lamp2 (Autodesk Fusion 360 design; units mm, degrees)
Autodesk Fusion 360 part; units mm, degrees
note: some values were not read from the file. Set by a fixed rule: which sketch regions a step uses.
sketch "Sketch1" plane through (0, 0, 0) normal (0, 0, 1) x (1, 0, 0)
  circle A0 centre (0, 0) radius 26
  circle A1 centre (0, 0) radius 16.5
  dimension "d1" = 52
  dimension "d2" = 33
  constraint coincident A0.centre A1.centre
  measures "d1" diameter of A0
  measures "d2" diameter of A1
extrude "Extrude1" add sketch "Sketch1" along normal blind 10 makes body 1
sketch "Sketch2" plane through (0, 0, 0) normal (0, 0, -1) x (1, 0, 0)
  circle A0 centre (0, 0) radius 16.5
  circle A1 centre (0, 0) radius 26
  circle A2 centre (0, 0) radius 20.5
  circle A3 centre (0, 0) radius 26
  dimension "d5" = 41
  constraint coincident A0.centre A1.centre
  constraint concentric A2 A3
  measures "d5" diameter of A2
extrude "Extrude2" add sketch "Sketch2" along normal blind 20 contours A1 A3 bodies 1
sketch "Sketch3" plane through (0, 0, -20) normal (0, 0, -1) x (1, 0, 0)
  circle A0 centre (0, 0) radius 20.5
  circle A1 centre (0, 0) radius 26
  circle A2 centre (0, 0) radius 26
  circle A3 centre (0, 0) radius 22
  dimension "d8" = 44
  constraint coincident A0.centre A1.centre
  constraint concentric A2 A3
  measures "d8" diameter of A3
extrude "Extrude3" add sketch "Sketch3" along normal blind 60 contours A1 A2 bodies 1
sketch "Sketch4" plane through (0, 0, 0) normal (0, 1, 0) x (1, 0, 0)
  circle A0 centre (0, 76) radius 4
  line L0 (0, 87) -> (0, 61.5698)
  line L1 (-16, 80) -> (14, 80)
  line L2 (-4, 76) -> (4, 76)
  line L3 (4, 76) -> (4, 83.4251)
  line L4 (4, 83.4251) -> (-4, 83.4251)
  line L5 (-4, 83.4251) -> (-4, 76)
  point P0 (0, 80)
  dimension "d11" = 8
  dimension "d12" = 8
  constraint vertical L0
  constraint horizontal L1
  constraint tangent A0 L1
  constraint coincident A0.centre L0
  constraint coincident L1 P0
  constraint coincident L0 P0
  constraint horizontal L2
  constraint vertical L3
  constraint horizontal L4
  constraint vertical L5
  constraint coincident A0.centre L2
  constraint coincident A0 L2.start
  measures "d11" diameter of A0
  measures "d12" distance of L2.start L2.end
extrude "Extrude4" cut sketch "Sketch4" along normal blind 70 bodies 1
sketch "Sketch5" plane through (0, 0, -80) normal (0, 0, -1) x (1, 0, 0)
  line L0 (-4, -25.6905) -> (-4, -21.6333)
  arc A0 (4, -21.6333) -> (-4, -21.6333) centre (0, 0) ccw
  line L1 (4, -21.6333) -> (4, -25.6905)
  arc A1 (4, -25.6905) -> (-4, -25.6905) centre (0, 0) ccw
  circle A2 centre (0, 0) radius 37.5
  circle A3 centre (0, 0) radius 26
  dimension "d15" = 75
  constraint coincident A0.centre A1.centre
  measures "d15" diameter of A2
extrude "Extrude5" add sketch "Sketch5" against normal blind 3 separate body makes body 2
